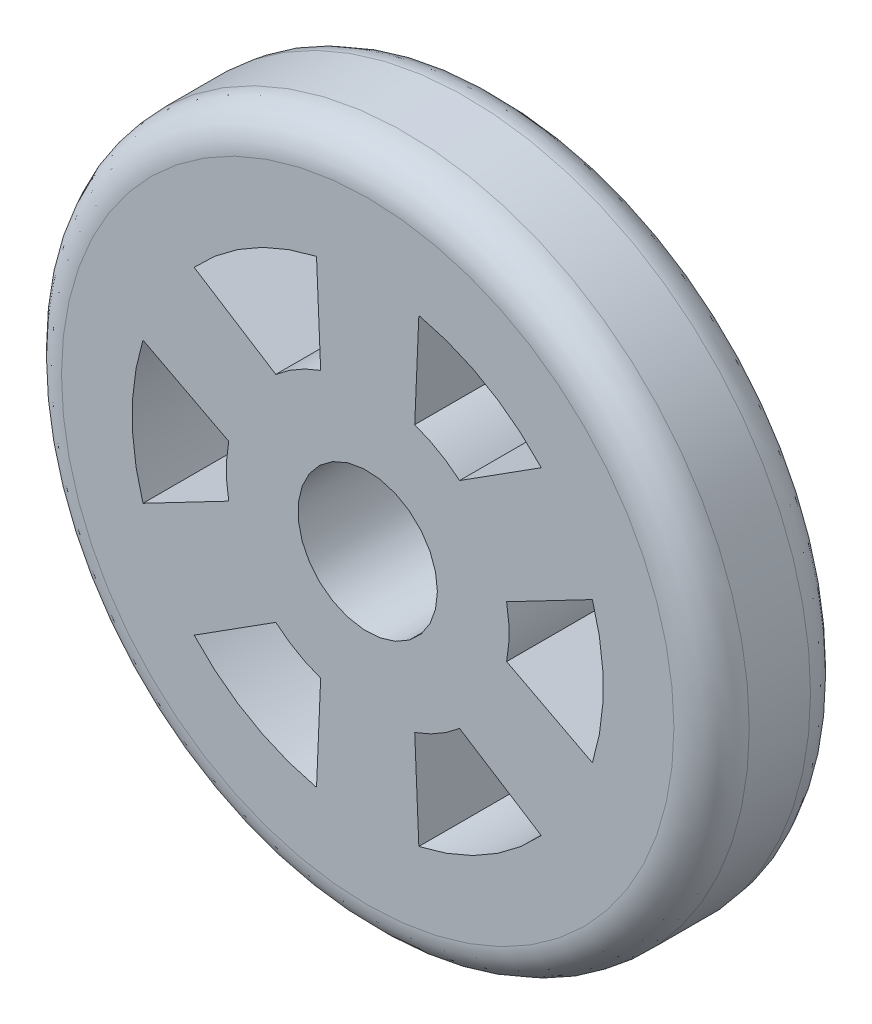
# Autodesk Inventor part: Wheel
Saved by Autodesk Inventor 2017 SP1 (Build 210196100, 196)
## iProperties
Created: 2018-03-03
Part Number: Wheel
Material: ABS Plastic
Document SubType Name: Modeling
Designer: Zach
Density: 1.06 g/cm^3
Appearance: Smooth - Black
Author: Zach
Autodesk Inventor part; units mm, degrees
ref_plane "YZ Plane" through (0, 0, 0) normal (1, 0, 0) x (0, 1, 0)
ref_plane "XZ Plane" through (0, 0, 0) normal (0, 1, 0) x (-1, 0, 0)
ref_plane "XY Plane" through (0, 0, 0) normal (0, 0, 1) x (1, 0, 0)
sketch "Sketch1" plane through (0, 0, 0) normal (0, 0, 1) x (1, 0, 0)
  circle A0 centre (0, 0) radius 73
  circle A1 centre (0, 0) radius 14.8
  circle A2 centre (0, 0) radius 50 construction
  circle A3 centre (0, 0) radius 30 construction
  arc A4 (47.697, -15) -> (47.697, 15) centre (0, 0) ccw
  arc A5 (29.4915, -5.5) -> (29.4915, 5.5) centre (0, 0) ccw
  line L0 (29.4915, 5.5) -> (47.697, 15)
  line L1 (29.4915, -5.5) -> (47.697, -15)
  arc A6 (36.8389, 33.8068) -> (10.8581, 48.8068) centre (0, 0) ccw
  arc A7 (19.5089, 22.7904) -> (9.9826, 28.2904) centre (0, 0) ccw
  line L2 (9.9826, 28.2904) -> (10.8581, 48.8068)
  line L3 (19.5089, 22.7904) -> (36.8389, 33.8068)
  arc A8 (-10.8581, 48.8068) -> (-36.8389, 33.8068) centre (0, 0) ccw
  arc A9 (-9.9826, 28.2904) -> (-19.5089, 22.7904) centre (0, 0) ccw
  line L4 (-19.5089, 22.7904) -> (-36.8389, 33.8068)
  line L5 (-9.9826, 28.2904) -> (-10.8581, 48.8068)
  arc A10 (-47.697, 15) -> (-47.697, -15) centre (0, 0) ccw
  arc A11 (-29.4915, 5.5) -> (-29.4915, -5.5) centre (0, 0) ccw
  line L6 (-29.4915, -5.5) -> (-47.697, -15)
  line L7 (-29.4915, 5.5) -> (-47.697, 15)
  arc A12 (-36.8389, -33.8068) -> (-10.8581, -48.8068) centre (0, 0) ccw
  arc A13 (-19.5089, -22.7904) -> (-9.9826, -28.2904) centre (0, 0) ccw
  line L8 (-9.9826, -28.2904) -> (-10.8581, -48.8068)
  line L9 (-19.5089, -22.7904) -> (-36.8389, -33.8068)
  arc A14 (10.8581, -48.8068) -> (36.8389, -33.8068) centre (0, 0) ccw
  arc A15 (9.9826, -28.2904) -> (19.5089, -22.7904) centre (0, 0) ccw
  line L10 (19.5089, -22.7904) -> (36.8389, -33.8068)
  line L11 (9.9826, -28.2904) -> (10.8581, -48.8068)
  point P0 (30, 0)
  point P1 (50, 0)
  point P2 (25, 43.3013)
  point P3 (15, 25.9808)
  point P4 (-25, 43.3013)
  point P5 (-15, 25.9808)
  point P6 (-50, 0)
  point P7 (-30, 0)
  point P8 (-25, -43.3013)
  point P9 (-15, -25.9808)
  point P10 (25, -43.3013)
  point P11 (15, -25.9808)
  dimension "d0" = 146
  dimension "d1" = 29.6
  dimension "d5" = 100
  dimension "d6" = 60
  dimension "d7" = 11
  dimension "d8" = 30
  dimension "d11" = 360
  constraints: 30 point on circle, 24 end point, 16 centre point, 4 coincident, 2 concentric, 2 horizontal alignment, 73 other
  measures "d0" diameter of A0
  measures "d1" diameter of A1
  measures "d5" diameter of A2
  measures "d6" diameter of A3
  measures "d7" distance of L1.start L0.start
  measures "d8" distance of L1.end L0.end
extrude "Extrusion1" add sketch "Sketch1" along normal mid plane 29
fillet "Fillet1" radius 8 2 edges at (-73, 0, 14.5) (-73, 0, -14.5)
body "Solid1"
